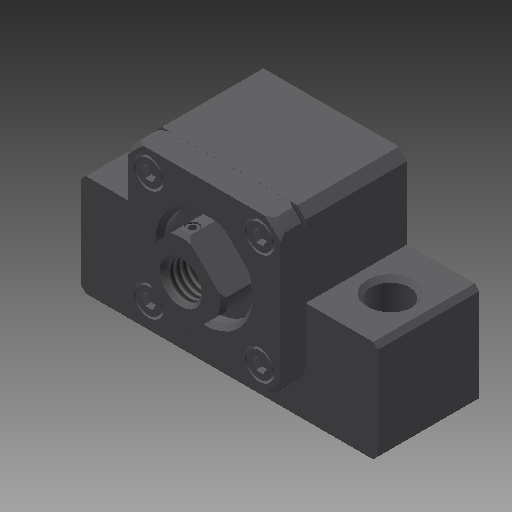
# Autodesk Inventor part: EK 10
Saved by Autodesk Inventor 2018 (Build 220112000, 112)
## iProperties
Category: PARTsolutions
Company: THK
Created: 2017-06-20
Part Number: EK 10
Catalog Web Link: www.cadenas.de
Description: Fixed Side type EK-
Vendor: THK
Document SubType Name: Modeling
Designer: psAdmin
Manufacturer: THK
Mass: 58.7713 g
Surface Area: 144.414 cm^2
Volume: 58.7713 cm^3
Density: 1 g/cm^3
Material: Generic
Appearance: PSOLRGB-192-192-192
PSOL_IDENT_0: {$CADENAS_DATA\23d-libs\thk\fed_screw\ball_screw\ball_screw_peripheral\suport_unit\fixed_side_type_e
PSOL_IDENT_1: k.prj},164 {VTYP=3D},{NB=EK 10},{LINA=EK 10},{NN=Fixed Side type EK},{DATE=02.06.2017 06:41:21},{GEO
PSOL_IDENT_2: MDATE=02.12.2016 13:20:00},{VERSION=},{LINEID=50},{LINESUBID=-1},{WBVAR=}  {NB=EK 10},{LINA=EK 10},{
PSOL_IDENT_3: KT=DUMMY},{IDNR=},{MN=EK 10},{SD=10.000},{L=24.000},{L1=6.000},{L2=29.500},{L3=6.000},{B=70.000},{H=
PSOL_IDENT_4: 43.000},{SB=35.000},{SH1=25.000},{B1=36.000},{H1=24.000},{P=52.000},{SD1=9.000},{SD2=0.000},{SH=0.00
PSOL_IDENT_5: 0},{NDM=3.000},{T=16.000},{SD3=14.500},{DV=1.000},{DK=23.000},{L4=8.500},{PCD=37.000},{D1=7.000},{WF=
PSOL_IDENT_6: 3.000},{WF1=1.500},{B2=0.000},{PCD1=48.000},{DB=21.000},{D=20.000},{R3=24.000}
NN: Fixed side type EK
NB: EK 10
NBSYN: $MN.
LINA: EK 10
MN: EK 10
SUPPLIER: THK
ARTICLENO: EK 10
BOMINFO: EK 10
CREATOR: CADENAS GmbH
Title: EK 10
Author: Cadenas PARTsolutions
Autodesk Inventor part; units mm, degrees
sketch "Sketch_1" plane through (0, 0, 0) normal (0, 0, 1) x (1, 0, 0)
  line L0 (-35, -23.92) -> (-33.92, -25)
  line L1 (-33.92, -25) -> (33.92, -25)
  line L2 (33.92, -25) -> (35, -23.92)
  line L3 (35, -23.92) -> (35, -2.08)
  line L4 (35, -2.08) -> (33.92, -1)
  line L5 (33.92, -1) -> (18, -1)
  line L6 (18, -1) -> (18, 16)
  line L7 (18, 16) -> (16, 18)
  line L8 (16, 18) -> (-16, 18)
  line L9 (-16, 18) -> (-18, 16)
  line L10 (-18, 16) -> (-18, -1)
  line L11 (-18, -1) -> (-33.92, -1)
  line L12 (-33.92, -1) -> (-35, -2.08)
  line L13 (-35, -2.08) -> (-35, -23.92)
  constraints: 28 end point
extrude "Extrusion1" add sketch "Sketch_1" against normal blind 24
sketch "Sketch_3" plane through (0, 0, -12) normal (0, 0, 1) x (1, 0, 0)
  line L0 (-26, -25) -> (-26, -1)
  line L1 (-26, -1) -> (-20.5, -1)
  line L2 (-20.5, -1) -> (-21.5, -2)
  line L3 (-21.5, -2) -> (-21.5, -24)
  line L4 (-21.5, -24) -> (-20.5, -25)
  line L5 (-20.5, -25) -> (-26, -25)
  line L6 (-26, -25) -> (-26, -1)
  constraints: 14 end point
revolve "Revolution1" cut sketch "Sketch_3" angle 360 about axis through (-26, -25, -12) along (0, -1, 0)
sketch "Sketch_4" plane through (0, 0, -12) normal (0, 0, 1) x (1, 0, 0)
  line L0 (26, -25) -> (26, -1)
  line L1 (26, -1) -> (31.5, -1)
  line L2 (31.5, -1) -> (30.5, -2)
  line L3 (30.5, -2) -> (30.5, -24)
  line L4 (30.5, -24) -> (31.5, -25)
  line L5 (31.5, -25) -> (26, -25)
  line L6 (26, -25) -> (26, -1)
  constraints: 14 end point
revolve "Revolution2" cut sketch "Sketch_4" angle 360 about axis through (26, -25, -12) along (0, -1, 0)
sketch "Sketch_17" plane through (0, 0, 0) normal (0, 0, 1) x (1, 0, 0)
  line L0 (-18, 18) -> (-18, -18)
  line L1 (-18, -18) -> (18, -18)
  line L2 (18, -18) -> (18, 18)
  line L3 (18, 18) -> (-18, 18)
  constraints: 8 end point
extrude "Extrusion2" add sketch "Sketch_17" along normal blind 3
sketch "Sketch_19" plane through (0, 0, 0) normal (1, 0, 0) x (0, 1, 0)
  line L0 (0, 3) -> (0, 11.5)
  line L1 (0, 11.5) -> (10, 11.5)
  line L2 (10, 11.5) -> (10, 4)
  line L3 (10, 4) -> (7, 4)
  line L4 (7, 4) -> (7, 3.5)
  line L5 (7, 3.5) -> (6, 3.5)
  line L6 (6, 3.5) -> (6, 3)
  line L7 (6, 3) -> (0, 3)
  line L8 (0, 3) -> (0, 11.5)
  constraints: 18 end point
revolve "Revolution3" add sketch "Sketch_19" angle 360 about axis through (0, 0, 3) along (0, 0, -1)
sketch "Sketch_18" plane through (0, 0, 11.5) normal (0, 0, 1) x (1, 0, 0)
  line L0 (-16, 16) -> (-16, -16)
  line L1 (-16, -16) -> (16, -16)
  line L2 (16, -16) -> (16, 16)
  line L3 (16, 16) -> (-16, 16)
  line L4 (-11.3137, 0) -> (0, -11.3137)
  line L5 (0, -11.3137) -> (11.3137, 0)
  line L6 (11.3137, 0) -> (0, 11.3137)
  line L7 (0, 11.3137) -> (-11.3137, 0)
  constraints: 16 end point
extrude "Extrusion3" cut sketch "Sketch_18" against normal blind 8.5
sketch "Sketch_20" plane through (0, 0, 3) normal (0, 0, 1) x (1, 0, 0)
  line L0 (-18, 18) -> (-18, -18)
  line L1 (-18, -18) -> (18, -18)
  line L2 (18, -18) -> (18, 18)
  line L3 (18, 18) -> (-18, 18)
  circle A0 centre (0, 0) radius 10.5
  constraints: 8 end point, 1 centre point
extrude "Extrusion4" add sketch "Sketch_20" along normal blind 3
sketch "Sketch_21" plane through (0, 0, 0) normal (1, 0, 0) x (0, 1, 0)
  line L0 (0, -50) -> (0, 50)
  line L1 (11.5, 6) -> (10.5, 6)
  line L2 (10.5, 6) -> (10.5, 5)
  line L3 (10.5, 5) -> (11.5, 6)
  constraints: 8 end point
revolve "Revolution4" cut sketch "Sketch_21" angle 360 about axis through (0, 0, -50) along (0, 0, -1)
sketch "Sketch_22" plane through (0, 0, 0) normal (1, 0, 0) x (0, 1, 0)
  line L0 (0, 3.5) -> (0, 11.5)
  line L1 (0, 11.5) -> (5, 11.5)
  line L2 (5, 11.5) -> (4.188, 10.688)
  line L3 (4.188, 10.688) -> (4.188, 4.312)
  line L4 (4.188, 4.312) -> (5, 3.5)
  line L5 (5, 3.5) -> (0, 3.5)
  line L6 (0, 3.5) -> (0, 11.5)
  constraints: 14 end point
revolve "Revolution5" cut sketch "Sketch_22" angle 360 about axis through (0, 0, 3.5) along (0, 0, -1)
thread "Thread1" size "M10x1.5" class "6H" standard "ISO Metric profile" full length
sketch "Sketch_24" plane through (0, 0, 0) normal (0.7071068, -0.7071068, 0) x (0, 0, -1)
  line L0 (-3, 18.5) -> (-6, 18.5)
  line L1 (-6, 18.5) -> (-6, 22)
  line L2 (-6, 22) -> (-3, 22)
  line L3 (-3, 22) -> (-3, 18.5)
  line L4 (-3, 18.5) -> (-6, 18.5)
  constraints: 10 end point
revolve "Revolution6" cut sketch "Sketch_24" angle 360 about axis through (13.0815, 13.0815, 3) along (0, 0, -1)
sketch "Sketch_25" plane through (0, 0, 0) normal (0.7071068, -0.7071068, 0) x (0, 0, -1)
  line L0 (-3, 18.5) -> (-6, 18.5)
  line L1 (-6, 18.5) -> (-6, 21.5)
  line L2 (-6, 21.5) -> (-3, 21.5)
  line L3 (-3, 21.5) -> (-3, 18.5)
  line L4 (-3, 18.5) -> (-6, 18.5)
  constraints: 10 end point
revolve "Revolution7" add sketch "Sketch_25" angle 360 about axis through (13.0815, 13.0815, 3) along (0, 0, -1)
sketch "Sketch_28" plane through (0, 0, 6) normal (0, 0, 1) x (0.7071068, 0.7071068, 0)
  line L0 (16.827, -0.4483) -> (18.0517, -1.673)
  line L1 (18.0517, -1.673) -> (19.7247, -1.2247)
  line L2 (19.7247, -1.2247) -> (20.173, 0.4483)
  line L3 (20.173, 0.4483) -> (18.9483, 1.673)
  line L4 (18.9483, 1.673) -> (17.2753, 1.2247)
  line L5 (17.2753, 1.2247) -> (16.827, -0.4483)
  constraints: 12 end point
extrude "Extrusion5" cut sketch "Sketch_28" along normal mid plane 3
pattern_linear "Rectangular Pattern1" count 2 spacing 26.163 along (-1, 0, 0) count 2 spacing 26.163 along (0, -1, 0) of "Revolution6"
pattern_linear "Rectangular Pattern2" count 2 spacing 26.163 along (-1, 0, 0) count 2 spacing 26.163 along (0, -1, 0) of "Revolution7"
pattern_linear "Rectangular Pattern3" count 2 spacing 26.163 along (-1, 0, 0) count 2 spacing 26.163 along (0, -1, 0) of "Extrusion5"
sketch "Sketch_30" plane through (0, 0, 0) normal (1, 0, 0) x (0, 1, 0)
  line L0 (0, -50) -> (0, 50)
  line L1 (9.2, 11.5) -> (10, 10.7)
  line L2 (10, 10.7) -> (10, 11.5)
  line L3 (10, 11.5) -> (9.2, 11.5)
  constraints: 8 end point
revolve "Revolution8" cut sketch "Sketch_30" angle 360 about axis through (0, 0, -50) along (0, 0, -1)
sketch "Sketch_31" plane through (0, 0, 0) normal (1, 0, 0) x (0, 1, 0)
  line L0 (0, -50) -> (0, 50)
  line L1 (10, 4.8) -> (9.2, 4)
  line L2 (9.2, 4) -> (10, 4)
  line L3 (10, 4) -> (10, 4.8)
  constraints: 8 end point
revolve "Revolution9" cut sketch "Sketch_31" angle 360 about axis through (0, 0, -50) along (0, 0, -1)
sketch "Sketch_32" plane through (0, 0, 0) normal (1, 0, 0) x (0, 1, 0)
  line L0 (10, 8.75) -> (5, 8.75)
  line L1 (5, 8.75) -> (5, 10.25)
  line L2 (5, 10.25) -> (10, 10.25)
  line L3 (10, 10.25) -> (10, 8.75)
  line L4 (10, 8.75) -> (5, 8.75)
  constraints: 10 end point
revolve "Revolution10" cut sketch "Sketch_32" angle 360 about axis through (0, 10, 8.75) along (0, 1, 0)
sketch "Sketch_33" plane through (0, 0, 0) normal (1, 0, 0) x (0, 1, 0)
  line L0 (9.8, 8.75) -> (6.8, 8.75)
  line L1 (6.8, 8.75) -> (6.8, 10.25)
  line L2 (6.8, 10.25) -> (9.5, 10.25)
  arc A0 (9.8, 9.95) -> (9.5, 10.25) centre (9.5, 9.95) ccw
  line L3 (9.8, 9.95) -> (9.8, 8.75)
  line L4 (9.8, 8.75) -> (6.8, 8.75)
  constraints: 10 end point, 2 point on circle, 1 centre point
revolve "Revolution11" add sketch "Sketch_33" angle 360 about axis through (0, 9.8, 8.75) along (0, 1, 0)
sketch "Sketch_34" plane through (0, 9.8, 0) normal (0, 1, 0) x (1, 0, 0)
  line L0 (-0.75, -9.183) -> (0, -9.616)
  line L1 (0, -9.616) -> (0.75, -9.183)
  line L2 (0.75, -9.183) -> (0.75, -8.317)
  line L3 (0.75, -8.317) -> (0, -7.884)
  line L4 (0, -7.884) -> (-0.75, -8.317)
  line L5 (-0.75, -8.317) -> (-0.75, -9.183)
  constraints: 12 end point
extrude "Extrusion6" cut sketch "Sketch_34" against normal blind 1.2
sketch "Sketch18" plane through (0, 0, -24) normal (0, 0, -1) x (-1, 0, 0)
  point P0 (0, 0)
hole "Hole1" at (0, 0, -24) direction (0, 0, 1) diameter 10 depth 27.5 counterbore diameter 14.5 counterbore depth 6
sketch "Sketch_55" plane through (0, 0, 0) normal (1, 0, 0) x (0, 1, 0)
  line L0 (0, -50) -> (0, 50)
  line L1 (10.55, -23.95) -> (10.5, -23.95)
  line L2 (10.5, -23.95) -> (10.5, -24)
  line L3 (10.5, -24) -> (10.55, -24)
  line L4 (10.55, -24) -> (10.55, -23.95)
  constraints: 10 end point
revolve "Revolution12" cut sketch "Sketch_55" angle 360 about axis through (0, 0, -50) along (0, 0, -1)
sketch "Sketch_16" plane through (0, 0, 0) normal (0, 0, 1) x (1, 0, 0)
  line L0 (-36, 36) -> (-36, -36)
  line L1 (-36, -36) -> (36, -36)
  line L2 (36, -36) -> (36, 36)
  line L3 (36, 36) -> (-36, 36)
  circle A0 centre (0, 0) radius 24
  constraints: 8 end point, 1 centre point
extrude "Extrusion7" cut sketch "Sketch_16" along normal blind 6
sketch "Sketch_35" plane through (0, 0, 0) normal (1, 0, 0) x (0, 1, 0)
  line L0 (0, -50) -> (0, 50)
  line L1 (23, 6) -> (24, 5)
  line L2 (24, 5) -> (24, 6)
  line L3 (24, 6) -> (23, 6)
  constraints: 8 end point
revolve "Revolution13" cut sketch "Sketch_35" angle 360 about axis through (0, 0, -50) along (0, 0, -1)
sketch "Sketch_50" plane through (0, 0, 0) normal (1, 0, 0) x (0, 1, 0)
  line L0 (0, -50) -> (0, 50)
  line L1 (24, 1) -> (23, 0)
  line L2 (23, 0) -> (24, 0)
  line L3 (24, 0) -> (24, 1)
  constraints: 8 end point
revolve "Revolution14" cut sketch "Sketch_50" angle 360 about axis through (0, 0, -50) along (0, 0, -1)
sketch "Sketch_51" plane through (0, 0, 0) normal (0, 0, 1) x (1, 0, 0)
  line L0 (-36, -36) -> (36, -36)
  line L1 (36, -36) -> (36, 36)
  line L2 (36, 36) -> (-36, 36)
  line L3 (-36, 36) -> (-36, -36)
  line L4 (-17.98, 17.98) -> (-17.98, -17.98)
  line L5 (-17.98, -17.98) -> (17.98, -17.98)
  line L6 (17.98, -17.98) -> (17.98, 17.98)
  line L7 (17.98, 17.98) -> (-17.98, 17.98)
  constraints: 16 end point
extrude "Extrusion8" cut sketch "Sketch_51" along normal blind 0.01
ref_plane "unit_XY" through (0, 0, 0) normal (0, 0, -1) x (1, 0, 0)
ref_plane "unit_YZ" through (0, 0, 0) normal (1, 0, 0) x (0, -1, 0)
ref_plane "unit_ZX" through (0, 0, 0) normal (0, -1, 0) x (0, 0, -1)
ref_plane "unit_collar_XY" through (0, 0, -18) normal (0, 0, 1) x (1, 0, 0)
ref_plane "unit_collar_YZ" through (0, 0, -18) normal (1, 0, 0) x (0, 1, 0)
ref_plane "unit_collar_ZX" through (0, 0, -18) normal (0, 1, 0) x (0, 0, 1)
body "Solid1"
